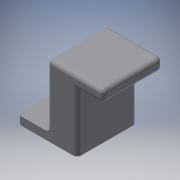
# Autodesk Inventor part: SwerveDriveClasp
Saved by Autodesk Inventor 2018 (Build 220112000, 112)
## iProperties
Created: 2018-10-19
Part Number: SwerveDriveClasp
Material: Generic
Document SubType Name: Modeling
Designer: reide
Density: 1 g/cm^3
Appearance: Default
Author: reide
Autodesk Inventor part; units mm, degrees
ref_plane "YZ Plane" through (0, 0, 0) normal (1, 0, 0) x (0, 1, 0)
ref_plane "XZ Plane" through (0, 0, 0) normal (0, 1, 0) x (-1, 0, 0)
ref_plane "XY Plane" through (0, 0, 0) normal (0, 0, 1) x (1, 0, 0)
sketch "Sketch1" plane through (0, 0, 0) normal (0, 0, 1) x (1, 0, 0)
  line L0 (0, 0) -> (15, 0)
  line L1 (15, 0) -> (15, 15)
  line L2 (15, 15) -> (0, 15)
  line L3 (0, 15) -> (0, 0)
  dimension "d0" = 15
  dimension "d1" = 15
  constraints: 8 end point, 2 parallel, 1 horizontal, 1 perpendicular
  measures "d0" distance of L1.end L2.end
  measures "d1" distance of L0.end L1.end
extrude "Extrusion1" add sketch "Sketch1" along normal blind 2
sketch "Sketch2" plane through (0, 0, 2) normal (0, 0, 1) x (1, 0, 0)
  line L0 (15, 0) -> (15, 15) projected
  line L1 (15, 15) -> (7.5, 15)
  line L2 (7.5, 15) -> (7.5, 0)
  line L3 (7.5, 0) -> (15, 0)
  line L4 (15, 0) -> (15, 15)
  point P0 (0, 0)
  dimension "d4" = 7.5
  constraints: 8 end point, 2 parallel, 1 horizontal, 1 perpendicular
  measures "d4" distance of L0.end L1.end
extrude "Extrusion2" add sketch "Sketch2" along normal blind 10.8
sketch "Sketch3" plane through (0, 0, 12.8) normal (0, 0, 1) x (1, 0, 0)
  line L0 (7.5, 15) -> (7.5, 0) projected
  line L1 (7.5, 15) -> (21.5, 15)
  line L2 (21.5, 15) -> (21.5, 0)
  line L3 (21.5, 0) -> (7.5, 0)
  line L4 (7.5, 0) -> (7.5, 15)
  point P0 (0, 0)
  dimension "d7" = 14
  constraints: 8 end point, 2 parallel, 1 horizontal, 1 perpendicular
  measures "d7" distance of L0.start L1.end
extrude "Extrusion3" add sketch "Sketch3" along normal blind 3
sketch "Sketch4" plane through (0, 0, 2) normal (0, 0, 1) x (1, 0, 0)
  line L0 (7.5, 0) -> (7.5, 15) projected
  line L1 (7.5, 15) -> (0, 15) projected
  line L2 (0, 15) -> (0, 0) projected
  line L3 (0, 0) -> (7.5, 0) projected
  line L4 (21.5, 15) -> (7.5, 15) projected
  line L5 (7.5, 15) -> (7.5, 0) projected
  line L6 (7.5, 0) -> (21.5, 0) projected
  line L7 (21.5, 0) -> (21.5, 15) projected
  line L8 (0, 15) -> (0, 0) projected
  line L9 (0, 7.5) -> (4, 7.5)
  circle A0 centre (4, 7.5) radius 1.25
  dimension "d10" = 4
  dimension "d11" = 2.5
  constraints: 2 end point, 1 centre point, 1 coincident, 1 horizontal, 1 midpoint
  measures "d10" distance of L9.start L9.end
  measures "d11" diameter of A0
extrude "Extrusion4" cut sketch "Sketch4" against normal blind 3 contours A0
fillet "Fillet1" radius 1 4 edges at (0, 0, 1) (0, 15, 1) (21.5, 0, 14.3) (21.5, 15, 14.3)
fillet "Fillet2" radius 1 9 edges at (21.2071, 0.2929, 15.8) (21.5, 7.5, 15.8) (21.2071, 14.7071, 15.8) (14, 15, 15.8) (14, 0, 15.8) (7.5, 0, 8.9) (7.5, 15, 8.9) (7.5, 7.5, 15.8) (7.5, 7.5, 2)
fillet "Fillet3" radius 1 7 edges at (15, 0, 6.4) (21.2071, 0.2929, 12.8) (21.5, 7.5, 12.8) (21.2071, 14.7071, 12.8) (17.75, 15, 12.8) (17.75, 0, 12.8) (15, 15, 6.4)
body "Solid1"
